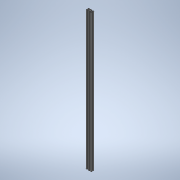
# Autodesk Inventor part: AP20x40x1000
Saved by Autodesk Inventor 2020 (Build 240168000, 168)
## iProperties
Created: 2016-10-26
Part Number: AP20x40x1000
Material: Типовые
Document SubType Name: Modeling
Designer: skhalipa
Density: 1 g/cm^3
Appearance: Анодированный — светло-серый
Author: skhalipa
Autodesk Inventor part; units mm, degrees
ref_plane "YZ Plane" through (0, 0, 0) normal (1, 0, 0) x (0, 1, 0)
ref_plane "XZ Plane" through (0, 0, 0) normal (0, 1, 0) x (-1, 0, 0)
ref_plane "XY Plane" through (0, 0, 0) normal (0, 0, 1) x (1, 0, 0)
sketch "Эскиз5" plane through (0, 0, 0) normal (0, 0, 1) x (1, 0, 0)
  line L0 (5.17, -0.2) -> (5.407, -0.042)
  line L1 (5.17, -0.2) -> (4.933, -0.042)
  arc A0 (4.933, -0.042) -> (4.7943, 0) centre (4.7943, -0.25) ccw
  line L2 (4.7943, 0) -> (0, 0)
  arc A1 (0, 0) -> (-0.1768, -0.0732) centre (0, -0.25) ccw
  line L3 (-0.1768, -0.0732) -> (-1.6768, -1.5732)
  arc A2 (-1.6768, -1.5732) -> (-1.5, -2) centre (-1.5, -1.75) ccw
  line L4 (-1.5, -2) -> (0.27, -2)
  arc A3 (0.47, -2.2) -> (0.27, -2) centre (0.27, -2.2) ccw
  line L5 (0.47, -2.2) -> (0.47, -3.013)
  arc A4 (0.1771, -3.7201) -> (0.47, -3.013) centre (-0.53, -3.013) ccw
  line L6 (0.1771, -3.7201) -> (-1.517, -5.4142)
  arc A5 (-2.9312, -6) -> (-1.517, -5.4142) centre (-2.9312, -4) ccw
  line L7 (-2.9312, -6) -> (-4.4923, -6)
  arc A6 (-4.4923, -6) -> (-4.6485, -6.0548) centre (-4.4923, -6.25) ccw
  line L8 (-4.6485, -6.0548) -> (-4.83, -6.2)
  line L9 (-5.0115, -6.0548) -> (-4.83, -6.2)
  arc A7 (-5.0115, -6.0548) -> (-5.1677, -6) centre (-5.1677, -6.25) ccw
  line L10 (-5.1677, -6) -> (-6.7288, -6)
  arc A8 (-8.143, -5.4142) -> (-6.7288, -6) centre (-6.7288, -4) ccw
  line L11 (-8.143, -5.4142) -> (-9.8371, -3.7201)
  arc A9 (-10.13, -3.013) -> (-9.8371, -3.7201) centre (-9.13, -3.013) ccw
  line L12 (-10.13, -3.013) -> (-10.13, -2.2)
  arc A10 (-9.93, -2) -> (-10.13, -2.2) centre (-9.93, -2.2) ccw
  line L13 (-9.93, -2) -> (-8.16, -2)
  arc A11 (-8.16, -2) -> (-7.9832, -1.5732) centre (-8.16, -1.75) ccw
  line L14 (-9.4832, -0.0732) -> (-7.9832, -1.5732)
  arc A12 (-9.4832, -0.0732) -> (-9.66, 0) centre (-9.66, -0.25) ccw
  line L15 (-9.66, 0) -> (-13.33, 0)
  arc A13 (-13.33, 0) -> (-14.83, -1.5) centre (-13.33, -1.5) ccw
  line L16 (-14.83, -5.17) -> (-14.83, -1.5)
  arc A14 (-14.83, -5.17) -> (-14.7568, -5.3468) centre (-14.58, -5.17) ccw
  line L17 (-14.7568, -5.3468) -> (-13.2568, -6.8468)
  arc A15 (-13.2568, -6.8468) -> (-12.83, -6.67) centre (-13.08, -6.67) ccw
  line L18 (-12.83, -4.9) -> (-12.83, -6.67)
  arc A16 (-12.63, -4.7) -> (-12.83, -4.9) centre (-12.63, -4.9) ccw
  line L19 (-11.817, -4.7) -> (-12.63, -4.7)
  arc A17 (-11.1099, -4.9929) -> (-11.817, -4.7) centre (-11.817, -5.7) ccw
  line L20 (-9.4158, -6.687) -> (-11.1099, -4.9929)
  arc A18 (-8.83, -8.1012) -> (-9.4158, -6.687) centre (-10.83, -8.1012) ccw
  line L21 (-8.83, -9.6623) -> (-8.83, -8.1012)
  arc A19 (-8.83, -9.6623) -> (-8.7752, -9.8185) centre (-8.58, -9.6623) ccw
  line L22 (-8.7752, -9.8185) -> (-8.63, -10)
  line L23 (-8.7752, -10.1815) -> (-8.63, -10)
  arc A20 (-8.7752, -10.1815) -> (-8.83, -10.3377) centre (-8.58, -10.3377) ccw
  line L24 (-8.83, -10.3377) -> (-8.83, -11.8988)
  arc A21 (-9.4158, -13.313) -> (-8.83, -11.8988) centre (-10.83, -11.8988) ccw
  line L25 (-9.4158, -13.313) -> (-11.1099, -15.0071)
  arc A22 (-11.817, -15.3) -> (-11.1099, -15.0071) centre (-11.817, -14.3) ccw
  line L26 (-11.817, -15.3) -> (-12.63, -15.3)
  arc A23 (-12.83, -15.1) -> (-12.63, -15.3) centre (-12.63, -15.1) ccw
  line L27 (-12.83, -15.1) -> (-12.83, -13.33)
  arc A24 (-12.83, -13.33) -> (-13.2568, -13.1532) centre (-13.08, -13.33) ccw
  line L28 (-14.7568, -14.6532) -> (-13.2568, -13.1532)
  arc A25 (-14.7568, -14.6532) -> (-14.83, -14.83) centre (-14.58, -14.83) ccw
  line L29 (-14.83, -14.83) -> (-14.83, -18.5)
  arc A26 (-14.83, -18.5) -> (-13.33, -20) centre (-13.33, -18.5) ccw
  line L30 (-9.66, -20) -> (-13.33, -20)
  arc A27 (-9.66, -20) -> (-9.4832, -19.9268) centre (-9.66, -19.75) ccw
  line L31 (-9.4832, -19.9268) -> (-7.9832, -18.4268)
  arc A28 (-7.9832, -18.4268) -> (-8.16, -18) centre (-8.16, -18.25) ccw
  line L32 (-9.93, -18) -> (-8.16, -18)
  arc A29 (-10.13, -17.8) -> (-9.93, -18) centre (-9.93, -17.8) ccw
  line L33 (-10.13, -16.987) -> (-10.13, -17.8)
  arc A30 (-9.8371, -16.2799) -> (-10.13, -16.987) centre (-9.13, -16.987) ccw
  line L34 (-8.143, -14.5858) -> (-9.8371, -16.2799)
  arc A31 (-6.7288, -14) -> (-8.143, -14.5858) centre (-6.7288, -16) ccw
  line L35 (-5.1677, -14) -> (-6.7288, -14)
  arc A32 (-5.1677, -14) -> (-5.0115, -13.9452) centre (-5.1677, -13.75) ccw
  line L36 (-5.0115, -13.9452) -> (-4.83, -13.8)
  line L37 (-4.6485, -13.9452) -> (-4.83, -13.8)
  arc A33 (-4.6485, -13.9452) -> (-4.4923, -14) centre (-4.4923, -13.75) ccw
  line L38 (-2.9312, -14) -> (-4.4923, -14)
  arc A34 (-1.517, -14.5858) -> (-2.9312, -14) centre (-2.9312, -16) ccw
  line L39 (0.1771, -16.2799) -> (-1.517, -14.5858)
  arc A35 (0.47, -16.987) -> (0.1771, -16.2799) centre (-0.53, -16.987) ccw
  line L40 (0.47, -17.8) -> (0.47, -16.987)
  arc A36 (0.27, -18) -> (0.47, -17.8) centre (0.27, -17.8) ccw
  line L41 (-1.5, -18) -> (0.27, -18)
  arc A37 (-1.5, -18) -> (-1.6768, -18.4268) centre (-1.5, -18.25) ccw
  line L42 (-0.1768, -19.9268) -> (-1.6768, -18.4268)
  arc A38 (-0.1768, -19.9268) -> (0, -20) centre (0, -19.75) ccw
  line L43 (4.7943, -20) -> (0, -20)
  arc A39 (4.7943, -20) -> (4.933, -19.958) centre (4.7943, -19.75) ccw
  line L44 (5.17, -19.8) -> (4.933, -19.958)
  line L45 (5.17, -19.8) -> (5.407, -19.958)
  arc A40 (5.407, -19.958) -> (5.5457, -20) centre (5.5457, -19.75) ccw
  line L46 (5.5457, -20) -> (10.34, -20)
  arc A41 (10.34, -20) -> (10.5168, -19.9268) centre (10.34, -19.75) ccw
  line L47 (10.5168, -19.9268) -> (12.0168, -18.4268)
  arc A42 (12.0168, -18.4268) -> (11.84, -18) centre (11.84, -18.25) ccw
  line L48 (11.84, -18) -> (10.07, -18)
  arc A43 (9.87, -17.8) -> (10.07, -18) centre (10.07, -17.8) ccw
  line L49 (9.87, -17.8) -> (9.87, -16.987)
  arc A44 (10.1629, -16.2799) -> (9.87, -16.987) centre (10.87, -16.987) ccw
  line L50 (10.1629, -16.2799) -> (11.857, -14.5858)
  arc A45 (13.2712, -14) -> (11.857, -14.5858) centre (13.2712, -16) ccw
  line L51 (13.2712, -14) -> (14.8323, -14)
  arc A46 (14.8323, -14) -> (14.9885, -13.9452) centre (14.8323, -13.75) ccw
  line L52 (14.9885, -13.9452) -> (15.17, -13.8)
  line L53 (15.3515, -13.9452) -> (15.17, -13.8)
  arc A47 (15.3515, -13.9452) -> (15.5077, -14) centre (15.5077, -13.75) ccw
  line L54 (15.5077, -14) -> (17.0688, -14)
  arc A48 (18.483, -14.5858) -> (17.0688, -14) centre (17.0688, -16) ccw
  line L55 (18.483, -14.5858) -> (20.1771, -16.2799)
  arc A49 (20.47, -16.987) -> (20.1771, -16.2799) centre (19.47, -16.987) ccw
  line L56 (20.47, -16.987) -> (20.47, -17.8)
  arc A50 (20.27, -18) -> (20.47, -17.8) centre (20.27, -17.8) ccw
  line L57 (20.27, -18) -> (18.5, -18)
  arc A51 (18.5, -18) -> (18.3232, -18.4268) centre (18.5, -18.25) ccw
  line L58 (19.8232, -19.9268) -> (18.3232, -18.4268)
  arc A52 (19.8232, -19.9268) -> (20, -20) centre (20, -19.75) ccw
  line L59 (20, -20) -> (23.67, -20)
  arc A53 (23.67, -20) -> (25.17, -18.5) centre (23.67, -18.5) ccw
  line L60 (25.17, -14.83) -> (25.17, -18.5)
  arc A54 (25.17, -14.83) -> (25.0968, -14.6532) centre (24.92, -14.83) ccw
  line L61 (25.0968, -14.6532) -> (23.5968, -13.1532)
  arc A55 (23.5968, -13.1532) -> (23.17, -13.33) centre (23.42, -13.33) ccw
  line L62 (23.17, -15.1) -> (23.17, -13.33)
  arc A56 (22.97, -15.3) -> (23.17, -15.1) centre (22.97, -15.1) ccw
  line L63 (22.157, -15.3) -> (22.97, -15.3)
  arc A57 (21.4499, -15.0071) -> (22.157, -15.3) centre (22.157, -14.3) ccw
  line L64 (19.7558, -13.313) -> (21.4499, -15.0071)
  arc A58 (19.17, -11.8988) -> (19.7558, -13.313) centre (21.17, -11.8988) ccw
  line L65 (19.17, -10.3377) -> (19.17, -11.8988)
  arc A59 (19.17, -10.3377) -> (19.1152, -10.1815) centre (18.92, -10.3377) ccw
  line L66 (19.1152, -10.1815) -> (18.97, -10)
  line L67 (19.1152, -9.8185) -> (18.97, -10)
  arc A60 (19.1152, -9.8185) -> (19.17, -9.6623) centre (18.92, -9.6623) ccw
  line L68 (19.17, -9.6623) -> (19.17, -8.1012)
  arc A61 (19.7558, -6.687) -> (19.17, -8.1012) centre (21.17, -8.1012) ccw
  line L69 (19.7558, -6.687) -> (21.4499, -4.9929)
  arc A62 (22.157, -4.7) -> (21.4499, -4.9929) centre (22.157, -5.7) ccw
  line L70 (22.157, -4.7) -> (22.97, -4.7)
  arc A63 (23.17, -4.9) -> (22.97, -4.7) centre (22.97, -4.9) ccw
  line L71 (23.17, -4.9) -> (23.17, -6.67)
  arc A64 (23.17, -6.67) -> (23.5968, -6.8468) centre (23.42, -6.67) ccw
  line L72 (25.0968, -5.3468) -> (23.5968, -6.8468)
  arc A65 (25.0968, -5.3468) -> (25.17, -5.17) centre (24.92, -5.17) ccw
  line L73 (25.17, -5.17) -> (25.17, -1.5)
  arc A66 (25.17, -1.5) -> (23.67, 0) centre (23.67, -1.5) ccw
  line L74 (20, 0) -> (23.67, 0)
  arc A67 (20, 0) -> (19.8232, -0.0732) centre (20, -0.25) ccw
  line L75 (19.8232, -0.0732) -> (18.3232, -1.5732)
  arc A68 (18.3232, -1.5732) -> (18.5, -2) centre (18.5, -1.75) ccw
  line L76 (20.27, -2) -> (18.5, -2)
  arc A69 (20.47, -2.2) -> (20.27, -2) centre (20.27, -2.2) ccw
  line L77 (20.47, -3.013) -> (20.47, -2.2)
  arc A70 (20.1771, -3.7201) -> (20.47, -3.013) centre (19.47, -3.013) ccw
  line L78 (18.483, -5.4142) -> (20.1771, -3.7201)
  arc A71 (17.0688, -6) -> (18.483, -5.4142) centre (17.0688, -4) ccw
  line L79 (15.5077, -6) -> (17.0688, -6)
  arc A72 (15.5077, -6) -> (15.3515, -6.0548) centre (15.5077, -6.25) ccw
  line L80 (15.3515, -6.0548) -> (15.17, -6.2)
  line L81 (14.9885, -6.0548) -> (15.17, -6.2)
  arc A73 (14.9885, -6.0548) -> (14.8323, -6) centre (14.8323, -6.25) ccw
  line L82 (13.2712, -6) -> (14.8323, -6)
  arc A74 (11.857, -5.4142) -> (13.2712, -6) centre (13.2712, -4) ccw
  line L83 (10.1629, -3.7201) -> (11.857, -5.4142)
  arc A75 (9.87, -3.013) -> (10.1629, -3.7201) centre (10.87, -3.013) ccw
  line L84 (9.87, -2.2) -> (9.87, -3.013)
  arc A76 (10.07, -2) -> (9.87, -2.2) centre (10.07, -2.2) ccw
  line L85 (11.84, -2) -> (10.07, -2)
  arc A77 (11.84, -2) -> (12.0168, -1.5732) centre (11.84, -1.75) ccw
  line L86 (10.5168, -0.0732) -> (12.0168, -1.5732)
  arc A78 (10.5168, -0.0732) -> (10.34, 0) centre (10.34, -0.25) ccw
  line L87 (5.5457, 0) -> (10.34, 0)
  arc A79 (5.5457, 0) -> (5.407, -0.042) centre (5.5457, -0.25) ccw
  line L88 (5.0227, -2) -> (5.3173, -2)
  arc A80 (6.3073, -2.4101) -> (5.3173, -2) centre (5.3173, -3.4) ccw
  line L89 (10.5842, -6.687) -> (6.3073, -2.4101)
  arc A81 (11.17, -8.1012) -> (10.5842, -6.687) centre (9.17, -8.1012) ccw
  line L90 (11.17, -11.8988) -> (11.17, -8.1012)
  arc A82 (10.5842, -13.313) -> (11.17, -11.8988) centre (9.17, -11.8988) ccw
  line L91 (10.5842, -13.313) -> (6.3073, -17.5899)
  arc A83 (5.3173, -18) -> (6.3073, -17.5899) centre (5.3173, -16.6) ccw
  line L92 (5.0227, -18) -> (5.3173, -18)
  arc A84 (4.0327, -17.5899) -> (5.0227, -18) centre (5.0227, -16.6) ccw
  line L93 (-0.2442, -13.313) -> (4.0327, -17.5899)
  arc A85 (-0.83, -11.8988) -> (-0.2442, -13.313) centre (1.17, -11.8988) ccw
  line L94 (-0.83, -11.8988) -> (-0.83, -8.1012)
  arc A86 (-0.2442, -6.687) -> (-0.83, -8.1012) centre (1.17, -8.1012) ccw
  line L95 (-0.2442, -6.687) -> (4.0327, -2.4101)
  arc A87 (5.0227, -2) -> (4.0327, -2.4101) centre (5.0227, -3.4) ccw
  circle A88 centre (-4.83, -10) radius 2.5
  circle A89 centre (15.17, -10) radius 2.5
  dimension "d214" = 0.25
  dimension "d215" = 1.5
  dimension "d216" = 0.2
  dimension "d217" = 1
  dimension "d218" = 2
  dimension "d219" = 5
  dimension "d220" = 1.4
  dimension "d221" = 135
  dimension "d222" = 90
  dimension "d223" = 90
  dimension "d224" = 38.66
  dimension "d225" = 38.66
  dimension "d226" = 90
  dimension "d227" = 90
  dimension "d228" = 90
  dimension "d229" = 90
  dimension "d230" = 45
  dimension "d231" = 45
  dimension "d232" = 90
  dimension "d233" = 90
  dimension "d234" = 56.31
  dimension "d235" = 56.31
  dimension "d236" = 90
  dimension "d237" = 90
  dimension "d238" = 90
  dimension "d239" = 90
  dimension "d240" = 90
  dimension "d241" = 90
  dimension "d242" = 45
  dimension "d243" = 45
  dimension "d244" = 2
  dimension "d245" = 4.7
  dimension "d246" = 14
  dimension "d247" = 15.3
  dimension "d248" = 24.7
  dimension "d249" = 26
  dimension "d250" = 34
  dimension "d251" = 35.3
  dimension "d252" = 40
  dimension "d253" = 7.4579
  dimension "d254" = 2.829
  dimension "d255" = 4.629
  dimension "d256" = 18.7711
  dimension "d257" = 21.6001
  dimension "d258" = 16.9711
  dimension "d259" = 14.1421
  dimension "d260" = 7.4579
  dimension "d261" = 2.829
  dimension "d262" = 4.629
  dimension "d263" = 18.7711
  dimension "d264" = 21.6001
  dimension "d265" = 16.9711
  dimension "d266" = 14.1421
  dimension "d267" = 10.6
  dimension "d268" = 4.7
  dimension "d269" = 15.3
  dimension "d270" = 1.3
  dimension "d271" = 9.3
  dimension "d272" = 21.552
  dimension "d273" = 21.552
  dimension "d274" = 5.9346
  dimension "d275" = 12.4939
  dimension "d276" = 6.5593
  dimension "d277" = 5.9346
  constraints: 240 tangent, 192 end point, 176 point on circle, 90 centre point, 75 equal radius, 42 parallel, 3 perpendicular, 1 horizontal, 1 vertical
  measures "d214" radius of A65
  measures "d215" radius of A66
  measures "d216" radius of A63
  measures "d217" radius of A62
  measures "d218" radius of A61
  measures "d219" diameter of A89
  measures "d220" radius of A80
  measures "d221" angle of L73 L72
  measures "d222" angle of L76 L60
  measures "d223" angle of L57 L60
  measures "d224" angle of L67 L60
  measures "d225" angle of L73 L66
  measures "d226" angle of L82 L60
  measures "d227" angle of L51 L60
  measures "d228" angle of L85 L60
  measures "d229" angle of L48 L60
  measures "d230" angle of L47 L60
  measures "d231" angle of L50 L60
  measures "d232" angle of L87 L60
  measures "d233" angle of L46 L60
  measures "d234" angle of L73 L1
  measures "d235" angle of L0 L60
  measures "d236" angle of L2 L60
  measures "d237" angle of L43 L60
  measures "d238" angle of L4 L60
  measures "d239" angle of L41 L60
  measures "d240" angle of L7 L60
  measures "d241" angle of L38 L60
  measures "d242" angle of L25 L60
  measures "d243" angle of L28 L60
  measures "d244" distance between parallel lines of L60 L62
  measures "d245" distance between parallel lines of L60 L56
  measures "d246" distance between parallel lines of L60 L90
  measures "d247" distance between parallel lines of L60 L49
  measures "d248" distance between parallel lines of L60 L40
  measures "d249" distance between parallel lines of L60 L94
  measures "d250" distance between parallel lines of L60 L24
  measures "d251" distance between parallel lines of L60 L33
  measures "d252" distance between parallel lines of L60 L29
  measures "d253" distance between parallel lines of L75 L72
  measures "d254" distance between parallel lines of L72 L69
  measures "d255" distance between parallel lines of L72 L91
  measures "d256" distance between parallel lines of L72 L6
  measures "d257" distance between parallel lines of L72 L3
  measures "d258" distance between parallel lines of L72 L95
  measures "d259" distance between parallel lines of L72 L31
  measures "d260" distance between parallel lines of L58 L61
  measures "d261" distance between parallel lines of L61 L64
  measures "d262" distance between parallel lines of L61 L89
  measures "d263" distance between parallel lines of L61 L39
  measures "d264" distance between parallel lines of L61 L42
  measures "d265" distance between parallel lines of L61 L93
  measures "d266" distance between parallel lines of L61 L14
  measures "d267" distance between parallel lines of L70 L63
  measures "d268" distance between parallel lines of L70 L74
  measures "d269" distance between parallel lines of L70 L59
  measures "d270" distance between parallel lines of L70 L79
  measures "d271" distance between parallel lines of L70 L54
  measures "d272" distance between parallel lines of L67 L23
  measures "d273" distance between parallel lines of L66 L22
  measures "d274" distance between parallel lines of L80 L52
  measures "d275" distance between parallel lines of L80 L8
  measures "d276" distance between parallel lines of L80 L36
  measures "d277" distance between parallel lines of L81 L53
extrude "Выдавливание1" add sketch "Эскиз5" along normal mid plane 1000
